Autodesk Inventor part; units mm, degrees
(part 2 of 2)
  spline S27 degree 3 poles (-6.8794, 42.2876) (-6.8611, 42.277) (-6.8428, 42.2665) (-6.8244, 42.2562) (-6.7977, 42.2413) (-6.7709, 42.2265) (-6.744, 42.2121) (-6.7179, 42.1982) (-6.6917, 42.1845) (-6.6654, 42.171) (-6.6399, 42.158) (-6.6144, 42.1453) (-6.5887, 42.1329) (-6.5639, 42.1208) (-6.5389, 42.109) (-6.5139, 42.0975) (-6.4898, 42.0864) (-6.4655, 42.0755) (-6.4412, 42.0649) (-6.4178, 42.0547) (-6.3942, 42.0447) (-6.3706, 42.0349) (-6.3479, 42.0255) (-6.3251, 42.0164) (-6.3022, 42.0075) (-6.2803, 41.9989) (-6.2583, 41.9906) (-6.2362, 41.9825) (-6.215, 41.9747) (-6.1937, 41.9671) (-6.1724, 41.9598) (-6.152, 41.9528) (-6.1316, 41.946) (-6.1111, 41.9394) (-6.0915, 41.9331) (-6.0719, 41.9269) (-6.0522, 41.921) (-6.0335, 41.9154) (-6.0147, 41.91) (-5.9959, 41.9047) (-5.978, 41.8998) (-5.9601, 41.895) (-5.9422, 41.8904) (-5.9252, 41.886) (-5.9081, 41.8818) (-5.8911, 41.8778) (-5.875, 41.874) (-5.8588, 41.8703) (-5.8427, 41.8668) (-5.8275, 41.8636) (-5.8123, 41.8605) (-5.797, 41.8575) (-5.7827, 41.8547) (-5.7684, 41.8521) (-5.7541, 41.8496) (-5.7408, 41.8473) (-5.7274, 41.8451) (-5.7141, 41.8431) (-5.7017, 41.8412) (-5.6893, 41.8394) (-5.6768, 41.8378) (-5.6654, 41.8363) (-5.654, 41.8349) (-5.6425, 41.8336) (-5.6321, 41.8324) (-5.6216, 41.8313) (-5.6111, 41.8304) (-5.6016, 41.8295) (-5.5921, 41.8287) (-5.5826, 41.828) (-5.5741, 41.8274) (-5.5656, 41.8269) (-5.5571, 41.8265) (-5.5496, 41.8261) (-5.5421, 41.8258) (-5.5346, 41.8255) (-5.5231, 41.8252) (-5.5115, 41.825) (-5.5, 41.825) knots 0 0 0 0 0.043076 0.043076 0.043076 0.105506 0.105506 0.105506 0.165888 0.165888 0.165888 0.224224 0.224224 0.224224 0.280513 0.280513 0.280513 0.334755 0.334755 0.334755 0.38695 0.38695 0.38695 0.437099 0.437099 0.437099 0.4852 0.4852 0.4852 0.531254 0.531254 0.531254 0.575262 0.575262 0.575262 0.617223 0.617223 0.617223 0.657137 0.657137 0.657137 0.695004 0.695004 0.695004 0.730824 0.730824 0.730824 0.764598 0.764598 0.764598 0.796324 0.796324 0.796324 0.826004 0.826004 0.826004 0.853636 0.853636 0.853636 0.879222 0.879222 0.879222 0.902761 0.902761 0.902761 0.924253 0.924253 0.924253 0.943699 0.943699 0.943699 0.961097 0.961097 0.961097 0.976448 0.976448 0.976448 1 1 1 1
  line L41 (-5.5, 41.825) -> (-4.55, 41.825)
  line L42 (-4.55, 44.961) -> (-4.55, 46.5908)
  line L43 (-4.55, 46.5908) -> (-5.5, 46.5908)
  spline S28 degree 3 poles (-5.5, 46.5908) (-5.5115, 46.5908) (-5.5306, 46.5905) (-5.5581, 46.5893) (-5.5836, 46.5877) (-5.6121, 46.5854) (-5.6435, 46.5822) (-5.6779, 46.578) (-5.7151, 46.5726) (-5.7551, 46.5661) (-5.798, 46.5582) (-5.8437, 46.5489) (-5.8921, 46.5379) (-5.9432, 46.5253) (-5.9969, 46.5109) (-6.0532, 46.4946) (-6.1121, 46.4763) (-6.1734, 46.4558) (-6.2372, 46.4332) (-6.3033, 46.4081) (-6.3716, 46.3807) (-6.4422, 46.3507) (-6.5149, 46.3181) (-6.5897, 46.2827) (-6.6664, 46.2445) (-6.745, 46.2034) (-6.8162, 46.1644) (-6.8611, 46.1388) (-6.8794, 46.1282) knots 0 0 0 0 0.023552 0.038904 0.056302 0.075747 0.097239 0.120778 0.146364 0.173997 0.203676 0.235403 0.269176 0.304996 0.342863 0.382777 0.424738 0.468746 0.5148 0.562902 0.61305 0.665245 0.719487 0.775776 0.834112 0.894494 0.956924 1 1 1 1
  arc A14 (-6.8794, 46.1282) -> (-6.8794, 45.4236) centre (2.0124, 45.7759) ccw
  spline S29 degree 3 poles (-6.8794, 45.4236) (-6.8611, 45.413) (-6.8428, 45.4025) (-6.8244, 45.3922) (-6.7977, 45.3773) (-6.7709, 45.3625) (-6.744, 45.3481) (-6.7179, 45.3342) (-6.6917, 45.3205) (-6.6654, 45.307) (-6.6399, 45.294) (-6.6144, 45.2813) (-6.5887, 45.2689) (-6.5639, 45.2568) (-6.5389, 45.245) (-6.5139, 45.2335) (-6.4898, 45.2224) (-6.4655, 45.2115) (-6.4412, 45.2009) (-6.4178, 45.1907) (-6.3942, 45.1807) (-6.3706, 45.1709) (-6.3479, 45.1615) (-6.3251, 45.1524) (-6.3022, 45.1435) (-6.2803, 45.1349) (-6.2583, 45.1266) (-6.2362, 45.1185) (-6.215, 45.1107) (-6.1937, 45.1031) (-6.1724, 45.0958) (-6.152, 45.0888) (-6.1316, 45.082) (-6.1111, 45.0754) (-6.0915, 45.0691) (-6.0719, 45.0629) (-6.0522, 45.057) (-6.0335, 45.0514) (-6.0147, 45.046) (-5.9959, 45.0407) (-5.978, 45.0358) (-5.9601, 45.031) (-5.9422, 45.0264) (-5.9252, 45.022) (-5.9081, 45.0178) (-5.8911, 45.0138) (-5.875, 45.01) (-5.8588, 45.0063) (-5.8427, 45.0028) (-5.8275, 44.9996) (-5.8123, 44.9965) (-5.797, 44.9935) (-5.7827, 44.9907) (-5.7684, 44.9881) (-5.7541, 44.9856) (-5.7408, 44.9833) (-5.7274, 44.9811) (-5.7141, 44.9791) (-5.7017, 44.9772) (-5.6893, 44.9754) (-5.6768, 44.9738) (-5.6654, 44.9723) (-5.654, 44.9709) (-5.6425, 44.9696) (-5.6321, 44.9684) (-5.6216, 44.9673) (-5.6111, 44.9664) (-5.6016, 44.9655) (-5.5921, 44.9647) (-5.5826, 44.964) (-5.5741, 44.9634) (-5.5656, 44.9629) (-5.5571, 44.9625) (-5.5496, 44.9621) (-5.5421, 44.9618) (-5.5346, 44.9615) (-5.5231, 44.9612) (-5.5115, 44.961) (-5.5, 44.961) knots 0 0 0 0 0.043076 0.043076 0.043076 0.105506 0.105506 0.105506 0.165888 0.165888 0.165888 0.224224 0.224224 0.224224 0.280513 0.280513 0.280513 0.334755 0.334755 0.334755 0.38695 0.38695 0.38695 0.437099 0.437099 0.437099 0.4852 0.4852 0.4852 0.531254 0.531254 0.531254 0.575262 0.575262 0.575262 0.617223 0.617223 0.617223 0.657137 0.657137 0.657137 0.695004 0.695004 0.695004 0.730824 0.730824 0.730824 0.764598 0.764598 0.764598 0.796324 0.796324 0.796324 0.826004 0.826004 0.826004 0.853636 0.853636 0.853636 0.879222 0.879222 0.879222 0.902761 0.902761 0.902761 0.924253 0.924253 0.924253 0.943699 0.943699 0.943699 0.961097 0.961097 0.961097 0.976448 0.976448 0.976448 1 1 1 1
  line L44 (-5.5, 44.961) -> (-4.55, 44.961)
  line L45 (-4.55, 48.097) -> (-4.55, 49.7268)
  line L46 (-4.55, 49.7268) -> (-5.5, 49.7268)
  spline S30 degree 3 poles (-5.5, 49.7268) (-5.5115, 49.7268) (-5.5306, 49.7265) (-5.5581, 49.7253) (-5.5836, 49.7237) (-5.6121, 49.7214) (-5.6435, 49.7182) (-5.6779, 49.714) (-5.7151, 49.7086) (-5.7551, 49.7021) (-5.798, 49.6942) (-5.8437, 49.6849) (-5.8921, 49.6739) (-5.9432, 49.6613) (-5.9969, 49.6469) (-6.0532, 49.6306) (-6.1121, 49.6123) (-6.1734, 49.5918) (-6.2372, 49.5692) (-6.3033, 49.5441) (-6.3716, 49.5167) (-6.4422, 49.4867) (-6.5149, 49.4541) (-6.5897, 49.4187) (-6.6664, 49.3805) (-6.745, 49.3394) (-6.8162, 49.3004) (-6.8611, 49.2748) (-6.8794, 49.2642) knots 0 0 0 0 0.023552 0.038904 0.056302 0.075747 0.097239 0.120778 0.146364 0.173997 0.203676 0.235403 0.269176 0.304996 0.342863 0.382777 0.424738 0.468746 0.5148 0.562902 0.61305 0.665245 0.719487 0.775776 0.834112 0.894494 0.956924 1 1 1 1
  arc A15 (-6.8794, 49.2642) -> (-6.8794, 48.5596) centre (2.0124, 48.9119) ccw
  spline S31 degree 3 poles (-6.8794, 48.5596) (-6.8611, 48.549) (-6.8428, 48.5385) (-6.8244, 48.5282) (-6.7977, 48.5133) (-6.7709, 48.4985) (-6.744, 48.4841) (-6.7179, 48.4702) (-6.6917, 48.4565) (-6.6654, 48.443) (-6.6399, 48.43) (-6.6144, 48.4173) (-6.5887, 48.4049) (-6.5639, 48.3928) (-6.5389, 48.381) (-6.5139, 48.3695) (-6.4898, 48.3584) (-6.4655, 48.3475) (-6.4412, 48.3369) (-6.4178, 48.3267) (-6.3942, 48.3167) (-6.3706, 48.3069) (-6.3479, 48.2975) (-6.3251, 48.2884) (-6.3022, 48.2795) (-6.2803, 48.2709) (-6.2583, 48.2626) (-6.2362, 48.2545) (-6.215, 48.2467) (-6.1937, 48.2391) (-6.1724, 48.2318) (-6.152, 48.2248) (-6.1316, 48.218) (-6.1111, 48.2114) (-6.0915, 48.2051) (-6.0719, 48.1989) (-6.0522, 48.193) (-6.0335, 48.1874) (-6.0147, 48.182) (-5.9959, 48.1767) (-5.978, 48.1718) (-5.9601, 48.167) (-5.9422, 48.1624) (-5.9252, 48.158) (-5.9081, 48.1538) (-5.8911, 48.1498) (-5.875, 48.146) (-5.8588, 48.1423) (-5.8427, 48.1388) (-5.8275, 48.1356) (-5.8123, 48.1325) (-5.797, 48.1295) (-5.7827, 48.1267) (-5.7684, 48.1241) (-5.7541, 48.1216) (-5.7408, 48.1193) (-5.7274, 48.1171) (-5.7141, 48.1151) (-5.7017, 48.1132) (-5.6893, 48.1114) (-5.6768, 48.1098) (-5.6654, 48.1083) (-5.654, 48.1069) (-5.6425, 48.1056) (-5.6321, 48.1044) (-5.6216, 48.1033) (-5.6111, 48.1024) (-5.6016, 48.1015) (-5.5921, 48.1007) (-5.5826, 48.1) (-5.5741, 48.0994) (-5.5656, 48.0989) (-5.5571, 48.0985) (-5.5496, 48.0981) (-5.5421, 48.0978) (-5.5346, 48.0975) (-5.5231, 48.0972) (-5.5115, 48.097) (-5.5, 48.097) knots 0 0 0 0 0.043076 0.043076 0.043076 0.105506 0.105506 0.105506 0.165888 0.165888 0.165888 0.224224 0.224224 0.224224 0.280513 0.280513 0.280513 0.334755 0.334755 0.334755 0.38695 0.38695 0.38695 0.437099 0.437099 0.437099 0.4852 0.4852 0.4852 0.531254 0.531254 0.531254 0.575262 0.575262 0.575262 0.617223 0.617223 0.617223 0.657137 0.657137 0.657137 0.695004 0.695004 0.695004 0.730824 0.730824 0.730824 0.764598 0.764598 0.764598 0.796324 0.796324 0.796324 0.826004 0.826004 0.826004 0.853636 0.853636 0.853636 0.879222 0.879222 0.879222 0.902761 0.902761 0.902761 0.924253 0.924253 0.924253 0.943699 0.943699 0.943699 0.961097 0.961097 0.961097 0.976448 0.976448 0.976448 1 1 1 1
  line L47 (-5.5, 48.097) -> (-4.55, 48.097)
  line L48 (-4.55, 51.233) -> (-4.55, 52.8628)
  line L49 (-4.55, 52.8628) -> (-5.5, 52.8628)
  spline S32 degree 3 poles (-5.5, 52.8628) (-5.5115, 52.8628) (-5.5306, 52.8625) (-5.5581, 52.8613) (-5.5836, 52.8597) (-5.6121, 52.8574) (-5.6435, 52.8542) (-5.6779, 52.85) (-5.7151, 52.8446) (-5.7551, 52.8381) (-5.798, 52.8302) (-5.8437, 52.8209) (-5.8921, 52.8099) (-5.9432, 52.7973) (-5.9969, 52.7829) (-6.0532, 52.7666) (-6.1121, 52.7483) (-6.1734, 52.7278) (-6.2372, 52.7052) (-6.3033, 52.6801) (-6.3716, 52.6527) (-6.4422, 52.6227) (-6.5149, 52.5901) (-6.5897, 52.5547) (-6.6664, 52.5165) (-6.745, 52.4754) (-6.8162, 52.4364) (-6.8611, 52.4108) (-6.8794, 52.4002) knots 0 0 0 0 0.023552 0.038904 0.056302 0.075747 0.097239 0.120778 0.146364 0.173997 0.203676 0.235403 0.269176 0.304996 0.342863 0.382777 0.424738 0.468746 0.5148 0.562902 0.61305 0.665245 0.719487 0.775776 0.834112 0.894494 0.956924 1 1 1 1
  arc A16 (-6.8794, 52.4002) -> (-6.8794, 51.6956) centre (2.0124, 52.0479) ccw
  spline S33 degree 3 poles (-6.8794, 51.6956) (-6.8611, 51.685) (-6.8428, 51.6745) (-6.8244, 51.6642) (-6.7977, 51.6493) (-6.7709, 51.6345) (-6.744, 51.6201) (-6.7179, 51.6062) (-6.6917, 51.5925) (-6.6654, 51.579) (-6.6399, 51.566) (-6.6144, 51.5533) (-6.5887, 51.5409) (-6.5639, 51.5288) (-6.5389, 51.517) (-6.5139, 51.5055) (-6.4898, 51.4944) (-6.4655, 51.4835) (-6.4412, 51.4729) (-6.4178, 51.4627) (-6.3942, 51.4527) (-6.3706, 51.4429) (-6.3479, 51.4335) (-6.3251, 51.4244) (-6.3022, 51.4155) (-6.2803, 51.4069) (-6.2583, 51.3986) (-6.2362, 51.3905) (-6.215, 51.3827) (-6.1937, 51.3751) (-6.1724, 51.3678) (-6.152, 51.3608) (-6.1316, 51.354) (-6.1111, 51.3474) (-6.0915, 51.3411) (-6.0719, 51.3349) (-6.0522, 51.329) (-6.0335, 51.3234) (-6.0147, 51.318) (-5.9959, 51.3127) (-5.978, 51.3078) (-5.9601, 51.303) (-5.9422, 51.2984) (-5.9252, 51.294) (-5.9081, 51.2898) (-5.8911, 51.2858) (-5.875, 51.282) (-5.8588, 51.2783) (-5.8427, 51.2748) (-5.8275, 51.2716) (-5.8123, 51.2685) (-5.797, 51.2655) (-5.7827, 51.2627) (-5.7684, 51.2601) (-5.7541, 51.2576) (-5.7408, 51.2553) (-5.7274, 51.2531) (-5.7141, 51.2511) (-5.7017, 51.2492) (-5.6893, 51.2474) (-5.6768, 51.2458) (-5.6654, 51.2443) (-5.654, 51.2429) (-5.6425, 51.2416) (-5.6321, 51.2404) (-5.6216, 51.2393) (-5.6111, 51.2384) (-5.6016, 51.2375) (-5.5921, 51.2367) (-5.5826, 51.236) (-5.5741, 51.2354) (-5.5656, 51.2349) (-5.5571, 51.2345) (-5.5496, 51.2341) (-5.5421, 51.2338) (-5.5346, 51.2335) (-5.5231, 51.2332) (-5.5115, 51.233) (-5.5, 51.233) knots 0 0 0 0 0.043076 0.043076 0.043076 0.105506 0.105506 0.105506 0.165888 0.165888 0.165888 0.224224 0.224224 0.224224 0.280513 0.280513 0.280513 0.334755 0.334755 0.334755 0.38695 0.38695 0.38695 0.437099 0.437099 0.437099 0.4852 0.4852 0.4852 0.531254 0.531254 0.531254 0.575262 0.575262 0.575262 0.617223 0.617223 0.617223 0.657137 0.657137 0.657137 0.695004 0.695004 0.695004 0.730824 0.730824 0.730824 0.764598 0.764598 0.764598 0.796324 0.796324 0.796324 0.826004 0.826004 0.826004 0.853636 0.853636 0.853636 0.879222 0.879222 0.879222 0.902761 0.902761 0.902761 0.924253 0.924253 0.924253 0.943699 0.943699 0.943699 0.961097 0.961097 0.961097 0.976448 0.976448 0.976448 1 1 1 1
  line L50 (-5.5, 51.233) -> (-4.55, 51.233)
  line L51 (-4.55, 54.369) -> (-4.55, 55.9988)
  line L52 (-4.55, 55.9988) -> (-5.5, 55.9988)
  spline S34 degree 3 poles (-5.5, 55.9988) (-5.5115, 55.9988) (-5.5306, 55.9985) (-5.5581, 55.9973) (-5.5836, 55.9957) (-5.6121, 55.9934) (-5.6435, 55.9902) (-5.6779, 55.986) (-5.7151, 55.9806) (-5.7551, 55.9741) (-5.798, 55.9662) (-5.8437, 55.9569) (-5.8921, 55.9459) (-5.9432, 55.9333) (-5.9969, 55.9189) (-6.0532, 55.9026) (-6.1121, 55.8843) (-6.1734, 55.8638) (-6.2372, 55.8412) (-6.3033, 55.8161) (-6.3716, 55.7887) (-6.4422, 55.7587) (-6.5149, 55.7261) (-6.5897, 55.6907) (-6.6664, 55.6525) (-6.745, 55.6114) (-6.8162, 55.5724) (-6.8611, 55.5468) (-6.8794, 55.5362) knots 0 0 0 0 0.023552 0.038904 0.056302 0.075747 0.097239 0.120778 0.146364 0.173997 0.203676 0.235403 0.269176 0.304996 0.342863 0.382777 0.424738 0.468746 0.5148 0.562902 0.61305 0.665245 0.719487 0.775776 0.834112 0.894494 0.956924 1 1 1 1
  arc A17 (-6.8794, 55.5362) -> (-6.8794, 54.8316) centre (2.0124, 55.1839) ccw
  spline S35 degree 3 poles (-6.8794, 54.8316) (-6.8611, 54.821) (-6.8428, 54.8105) (-6.8244, 54.8002) (-6.7977, 54.7853) (-6.7709, 54.7705) (-6.744, 54.7561) (-6.7179, 54.7422) (-6.6917, 54.7285) (-6.6654, 54.715) (-6.6399, 54.702) (-6.6144, 54.6893) (-6.5887, 54.6769) (-6.5639, 54.6648) (-6.5389, 54.653) (-6.5139, 54.6415) (-6.4898, 54.6304) (-6.4655, 54.6195) (-6.4412, 54.6089) (-6.4178, 54.5987) (-6.3942, 54.5887) (-6.3706, 54.5789) (-6.3479, 54.5695) (-6.3251, 54.5604) (-6.3022, 54.5515) (-6.2803, 54.5429) (-6.2583, 54.5346) (-6.2362, 54.5265) (-6.215, 54.5187) (-6.1937, 54.5111) (-6.1724, 54.5038) (-6.152, 54.4968) (-6.1316, 54.49) (-6.1111, 54.4834) (-6.0915, 54.4771) (-6.0719, 54.4709) (-6.0522, 54.465) (-6.0335, 54.4594) (-6.0147, 54.454) (-5.9959, 54.4487) (-5.978, 54.4438) (-5.9601, 54.439) (-5.9422, 54.4344) (-5.9252, 54.43) (-5.9081, 54.4258) (-5.8911, 54.4218) (-5.875, 54.418) (-5.8588, 54.4143) (-5.8427, 54.4108) (-5.8275, 54.4076) (-5.8123, 54.4045) (-5.797, 54.4015) (-5.7827, 54.3987) (-5.7684, 54.3961) (-5.7541, 54.3936) (-5.7408, 54.3913) (-5.7274, 54.3891) (-5.7141, 54.3871) (-5.7017, 54.3852) (-5.6893, 54.3834) (-5.6768, 54.3818) (-5.6654, 54.3803) (-5.654, 54.3789) (-5.6425, 54.3776) (-5.6321, 54.3764) (-5.6216, 54.3753) (-5.6111, 54.3744) (-5.6016, 54.3735) (-5.5921, 54.3727) (-5.5826, 54.372) (-5.5741, 54.3714) (-5.5656, 54.3709) (-5.5571, 54.3705) (-5.5496, 54.3701) (-5.5421, 54.3698) (-5.5346, 54.3695) (-5.5231, 54.3692) (-5.5115, 54.369) (-5.5, 54.369) knots 0 0 0 0 0.043076 0.043076 0.043076 0.105506 0.105506 0.105506 0.165888 0.165888 0.165888 0.224224 0.224224 0.224224 0.280513 0.280513 0.280513 0.334755 0.334755 0.334755 0.38695 0.38695 0.38695 0.437099 0.437099 0.437099 0.4852 0.4852 0.4852 0.531254 0.531254 0.531254 0.575262 0.575262 0.575262 0.617223 0.617223 0.617223 0.657137 0.657137 0.657137 0.695004 0.695004 0.695004 0.730824 0.730824 0.730824 0.764598 0.764598 0.764598 0.796324 0.796324 0.796324 0.826004 0.826004 0.826004 0.853636 0.853636 0.853636 0.879222 0.879222 0.879222 0.902761 0.902761 0.902761 0.924253 0.924253 0.924253 0.943699 0.943699 0.943699 0.961097 0.961097 0.961097 0.976448 0.976448 0.976448 1 1 1 1
  line L53 (-5.5, 54.369) -> (-4.55, 54.369)
  line L54 (-4.55, 57.505) -> (-4.55, 59.1348)
  line L55 (-4.55, 59.1348) -> (-5.5, 59.1348)
  spline S36 degree 3 poles (-5.5, 59.1348) (-5.5115, 59.1348) (-5.5306, 59.1345) (-5.5581, 59.1333) (-5.5836, 59.1317) (-5.6121, 59.1294) (-5.6435, 59.1262) (-5.6779, 59.122) (-5.7151, 59.1166) (-5.7551, 59.1101) (-5.798, 59.1022) (-5.8437, 59.0929) (-5.8921, 59.0819) (-5.9432, 59.0693) (-5.9969, 59.0549) (-6.0532, 59.0386) (-6.1121, 59.0203) (-6.1734, 58.9998) (-6.2372, 58.9772) (-6.3033, 58.9521) (-6.3716, 58.9247) (-6.4422, 58.8947) (-6.5149, 58.8621) (-6.5897, 58.8267) (-6.6664, 58.7885) (-6.745, 58.7474) (-6.8162, 58.7084) (-6.8611, 58.6828) (-6.8794, 58.6722) knots 0 0 0 0 0.023552 0.038904 0.056302 0.075747 0.097239 0.120778 0.146364 0.173997 0.203676 0.235403 0.269176 0.304996 0.342863 0.382777 0.424738 0.468746 0.5148 0.562902 0.61305 0.665245 0.719487 0.775776 0.834112 0.894494 0.956924 1 1 1 1
  arc A18 (-6.8794, 58.6722) -> (-6.8794, 57.9676) centre (2.0124, 58.3199) ccw
  spline S37 degree 3 poles (-6.8794, 57.9676) (-6.8611, 57.957) (-6.8428, 57.9465) (-6.8244, 57.9362) (-6.7977, 57.9213) (-6.7709, 57.9065) (-6.744, 57.8921) (-6.7179, 57.8782) (-6.6917, 57.8645) (-6.6654, 57.851) (-6.6399, 57.838) (-6.6144, 57.8253) (-6.5887, 57.8129) (-6.5639, 57.8008) (-6.5389, 57.789) (-6.5139, 57.7775) (-6.4898, 57.7664) (-6.4655, 57.7555) (-6.4412, 57.7449) (-6.4178, 57.7347) (-6.3942, 57.7247) (-6.3706, 57.7149) (-6.3479, 57.7055) (-6.3251, 57.6964) (-6.3022, 57.6875) (-6.2803, 57.6789) (-6.2583, 57.6706) (-6.2362, 57.6625) (-6.215, 57.6547) (-6.1937, 57.6471) (-6.1724, 57.6398) (-6.152, 57.6328) (-6.1316, 57.626) (-6.1111, 57.6194) (-6.0915, 57.6131) (-6.0719, 57.6069) (-6.0522, 57.601) (-6.0335, 57.5954) (-6.0147, 57.59) (-5.9959, 57.5847) (-5.978, 57.5798) (-5.9601, 57.575) (-5.9422, 57.5704) (-5.9252, 57.566) (-5.9081, 57.5618) (-5.8911, 57.5578) (-5.875, 57.554) (-5.8588, 57.5503) (-5.8427, 57.5468) (-5.8275, 57.5436) (-5.8123, 57.5405) (-5.797, 57.5375) (-5.7827, 57.5347) (-5.7684, 57.5321) (-5.7541, 57.5296) (-5.7408, 57.5273) (-5.7274, 57.5251) (-5.7141, 57.5231) (-5.7017, 57.5212) (-5.6893, 57.5194) (-5.6768, 57.5178) (-5.6654, 57.5163) (-5.654, 57.5149) (-5.6425, 57.5136) (-5.6321, 57.5124) (-5.6216, 57.5113) (-5.6111, 57.5104) (-5.6016, 57.5095) (-5.5921, 57.5087) (-5.5826, 57.508) (-5.5741, 57.5074) (-5.5656, 57.5069) (-5.5571, 57.5065) (-5.5496, 57.5061) (-5.5421, 57.5058) (-5.5346, 57.5055) (-5.5231, 57.5052) (-5.5115, 57.505) (-5.5, 57.505) knots 0 0 0 0 0.043076 0.043076 0.043076 0.105506 0.105506 0.105506 0.165888 0.165888 0.165888 0.224224 0.224224 0.224224 0.280513 0.280513 0.280513 0.334755 0.334755 0.334755 0.38695 0.38695 0.38695 0.437099 0.437099 0.437099 0.4852 0.4852 0.4852 0.531254 0.531254 0.531254 0.575262 0.575262 0.575262 0.617223 0.617223 0.617223 0.657137 0.657137 0.657137 0.695004 0.695004 0.695004 0.730824 0.730824 0.730824 0.764598 0.764598 0.764598 0.796324 0.796324 0.796324 0.826004 0.826004 0.826004 0.853636 0.853636 0.853636 0.879222 0.879222 0.879222 0.902761 0.902761 0.902761 0.924253 0.924253 0.924253 0.943699 0.943699 0.943699 0.961097 0.961097 0.961097 0.976448 0.976448 0.976448 1 1 1 1
  line L56 (-5.5, 57.505) -> (-4.55, 57.505)
  line L57 (-4.55, 60.641) -> (-4.55, 62.2708)
  line L58 (-4.55, 62.2708) -> (-5.5, 62.2708)
  spline S38 degree 3 poles (-5.5, 62.2708) (-5.5115, 62.2708) (-5.5306, 62.2705) (-5.5581, 62.2693) (-5.5836, 62.2677) (-5.6121, 62.2654) (-5.6435, 62.2622) (-5.6779, 62.258) (-5.7151, 62.2526) (-5.7551, 62.2461) (-5.798, 62.2382) (-5.8437, 62.2289) (-5.8921, 62.2179) (-5.9432, 62.2053) (-5.9969, 62.1909) (-6.0532, 62.1746) (-6.1121, 62.1563) (-6.1734, 62.1358) (-6.2372, 62.1132) (-6.3033, 62.0881) (-6.3716, 62.0607) (-6.4422, 62.0307) (-6.5149, 61.9981) (-6.5897, 61.9627) (-6.6664, 61.9245) (-6.745, 61.8834) (-6.8162, 61.8444) (-6.8611, 61.8188) (-6.8794, 61.8082) knots 0 0 0 0 0.023552 0.038904 0.056302 0.075747 0.097239 0.120778 0.146364 0.173997 0.203676 0.235403 0.269176 0.304996 0.342863 0.382777 0.424738 0.468746 0.5148 0.562902 0.61305 0.665245 0.719487 0.775776 0.834112 0.894494 0.956924 1 1 1 1
  arc A19 (-6.8794, 61.8082) -> (-6.8794, 61.1036) centre (2.0124, 61.4559) ccw
  spline S39 degree 3 poles (-6.8794, 61.1036) (-6.8611, 61.093) (-6.8428, 61.0825) (-6.8244, 61.0722) (-6.7977, 61.0573) (-6.7709, 61.0425) (-6.744, 61.0281) (-6.7179, 61.0142) (-6.6917, 61.0005) (-6.6654, 60.987) (-6.6399, 60.974) (-6.6144, 60.9613) (-6.5887, 60.9489) (-6.5639, 60.9368) (-6.5389, 60.925) (-6.5139, 60.9135) (-6.4898, 60.9024) (-6.4655, 60.8915) (-6.4412, 60.8809) (-6.4178, 60.8707) (-6.3942, 60.8607) (-6.3706, 60.8509) (-6.3479, 60.8415) (-6.3251, 60.8324) (-6.3022, 60.8235) (-6.2803, 60.8149) (-6.2583, 60.8066) (-6.2362, 60.7985) (-6.215, 60.7907) (-6.1937, 60.7831) (-6.1724, 60.7758) (-6.152, 60.7688) (-6.1316, 60.762) (-6.1111, 60.7554) (-6.0915, 60.7491) (-6.0719, 60.7429) (-6.0522, 60.737) (-6.0335, 60.7314) (-6.0147, 60.726) (-5.9959, 60.7207) (-5.978, 60.7158) (-5.9601, 60.711) (-5.9422, 60.7064) (-5.9252, 60.702) (-5.9081, 60.6978) (-5.8911, 60.6938) (-5.875, 60.69) (-5.8588, 60.6863) (-5.8427, 60.6828) (-5.8275, 60.6796) (-5.8123, 60.6765) (-5.797, 60.6735) (-5.7827, 60.6707) (-5.7684, 60.6681) (-5.7541, 60.6656) (-5.7408, 60.6633) (-5.7274, 60.6611) (-5.7141, 60.6591) (-5.7017, 60.6572) (-5.6893, 60.6554) (-5.6768, 60.6538) (-5.6654, 60.6523) (-5.654, 60.6509) (-5.6425, 60.6496) (-5.6321, 60.6484) (-5.6216, 60.6473) (-5.6111, 60.6464) (-5.6016, 60.6455) (-5.5921, 60.6447) (-5.5826, 60.644) (-5.5741, 60.6434) (-5.5656, 60.6429) (-5.5571, 60.6425) (-5.5496, 60.6421) (-5.5421, 60.6418) (-5.5346, 60.6415) (-5.5231, 60.6412) (-5.5115, 60.641) (-5.5, 60.641) knots 0 0 0 0 0.043076 0.043076 0.043076 0.105506 0.105506 0.105506 0.165888 0.165888 0.165888 0.224224 0.224224 0.224224 0.280513 0.280513 0.280513 0.334755 0.334755 0.334755 0.38695 0.38695 0.38695 0.437099 0.437099 0.437099 0.4852 0.4852 0.4852 0.531254 0.531254 0.531254 0.575262 0.575262 0.575262 0.617223 0.617223 0.617223 0.657137 0.657137 0.657137 0.695004 0.695004 0.695004 0.730824 0.730824 0.730824 0.764598 0.764598 0.764598 0.796324 0.796324 0.796324 0.826004 0.826004 0.826004 0.853636 0.853636 0.853636 0.879222 0.879222 0.879222 0.902761 0.902761 0.902761 0.924253 0.924253 0.924253 0.943699 0.943699 0.943699 0.961097 0.961097 0.961097 0.976448 0.976448 0.976448 1 1 1 1
  line L59 (-5.5, 60.641) -> (-4.55, 60.641)
  line L60 (-4.55, 63.777) -> (-4.55, 65.4068)
  line L61 (-4.55, 65.4068) -> (-5.5, 65.4068)
  spline S40 degree 3 poles (-5.5, 65.4068) (-5.5115, 65.4068) (-5.5306, 65.4065) (-5.5581, 65.4053) (-5.5836, 65.4037) (-5.6121, 65.4014) (-5.6435, 65.3982) (-5.6779, 65.394) (-5.7151, 65.3886) (-5.7551, 65.3821) (-5.798, 65.3742) (-5.8437, 65.3649) (-5.8921, 65.3539) (-5.9432, 65.3413) (-5.9969, 65.3269) (-6.0532, 65.3106) (-6.1121, 65.2923) (-6.1734, 65.2718) (-6.2372, 65.2492) (-6.3033, 65.2241) (-6.3716, 65.1967) (-6.4422, 65.1667) (-6.5149, 65.1341) (-6.5897, 65.0987) (-6.6664, 65.0605) (-6.745, 65.0194) (-6.8162, 64.9804) (-6.8611, 64.9548) (-6.8794, 64.9442) knots 0 0 0 0 0.023552 0.038904 0.056302 0.075747 0.097239 0.120778 0.146364 0.173997 0.203676 0.235403 0.269176 0.304996 0.342863 0.382777 0.424738 0.468746 0.5148 0.562902 0.61305 0.665245 0.719487 0.775776 0.834112 0.894494 0.956924 1 1 1 1
  arc A20 (-6.8794, 64.9442) -> (-6.8794, 64.2396) centre (2.0124, 64.5919) ccw
  spline S41 degree 3 poles (-6.8794, 64.2396) (-6.8611, 64.229) (-6.8428, 64.2185) (-6.8244, 64.2082) (-6.7977, 64.1933) (-6.7709, 64.1785) (-6.744, 64.1641) (-6.7179, 64.1502) (-6.6917, 64.1365) (-6.6654, 64.123) (-6.6399, 64.11) (-6.6144, 64.0973) (-6.5887, 64.0849) (-6.5639, 64.0728) (-6.5389, 64.061) (-6.5139, 64.0495) (-6.4898, 64.0384) (-6.4655, 64.0275) (-6.4412, 64.0169) (-6.4178, 64.0067) (-6.3942, 63.9967) (-6.3706, 63.9869) (-6.3479, 63.9775) (-6.3251, 63.9684) (-6.3022, 63.9595) (-6.2803, 63.9509) (-6.2583, 63.9426) (-6.2362, 63.9345) (-6.215, 63.9267) (-6.1937, 63.9191) (-6.1724, 63.9118) (-6.152, 63.9048) (-6.1316, 63.898) (-6.1111, 63.8914) (-6.0915, 63.8851) (-6.0719, 63.8789) (-6.0522, 63.873) (-6.0335, 63.8674) (-6.0147, 63.862) (-5.9959, 63.8567) (-5.978, 63.8518) (-5.9601, 63.847) (-5.9422, 63.8424) (-5.9252, 63.838) (-5.9081, 63.8338) (-5.8911, 63.8298) (-5.875, 63.826) (-5.8588, 63.8223) (-5.8427, 63.8188) (-5.8275, 63.8156) (-5.8123, 63.8125) (-5.797, 63.8095) (-5.7827, 63.8067) (-5.7684, 63.8041) (-5.7541, 63.8016) (-5.7408, 63.7993) (-5.7274, 63.7971) (-5.7141, 63.7951) (-5.7017, 63.7932) (-5.6893, 63.7914) (-5.6768, 63.7898) (-5.6654, 63.7883) (-5.654, 63.7869) (-5.6425, 63.7856) (-5.6321, 63.7844) (-5.6216, 63.7833) (-5.6111, 63.7824) (-5.6016, 63.7815) (-5.5921, 63.7807) (-5.5826, 63.78) (-5.5741, 63.7794) (-5.5656, 63.7789) (-5.5571, 63.7785) (-5.5496, 63.7781) (-5.5421, 63.7778) (-5.5346, 63.7775) (-5.5231, 63.7772) (-5.5115, 63.777) (-5.5, 63.777) knots 0 0 0 0 0.043076 0.043076 0.043076 0.105506 0.105506 0.105506 0.165888 0.165888 0.165888 0.224224 0.224224 0.224224 0.280513 0.280513 0.280513 0.334755 0.334755 0.334755 0.38695 0.38695 0.38695 0.437099 0.437099 0.437099 0.4852 0.4852 0.4852 0.531254 0.531254 0.531254 0.575262 0.575262 0.575262 0.617223 0.617223 0.617223 0.657137 0.657137 0.657137 0.695004 0.695004 0.695004 0.730824 0.730824 0.730824 0.764598 0.764598 0.764598 0.796324 0.796324 0.796324 0.826004 0.826004 0.826004 0.853636 0.853636 0.853636 0.879222 0.879222 0.879222 0.902761 0.902761 0.902761 0.924253 0.924253 0.924253 0.943699 0.943699 0.943699 0.961097 0.961097 0.961097 0.976448 0.976448 0.976448 1 1 1 1
  line L62 (-5.5, 63.777) -> (-4.55, 63.777)
  line L63 (-4.55, 66.913) -> (-4.55, 68.5428)
  line L64 (-4.55, 68.5428) -> (-5.5, 68.5428)
  spline S42 degree 3 poles (-5.5, 68.5428) (-5.5115, 68.5428) (-5.5306, 68.5425) (-5.5581, 68.5413) (-5.5836, 68.5397) (-5.6121, 68.5374) (-5.6435, 68.5342) (-5.6779, 68.53) (-5.7151, 68.5246) (-5.7551, 68.5181) (-5.798, 68.5102) (-5.8437, 68.5009) (-5.8921, 68.4899) (-5.9432, 68.4773) (-5.9969, 68.4629) (-6.0532, 68.4466) (-6.1121, 68.4283) (-6.1734, 68.4078) (-6.2372, 68.3852) (-6.3033, 68.3601) (-6.3716, 68.3327) (-6.4422, 68.3027) (-6.5149, 68.2701) (-6.5897, 68.2347) (-6.6664, 68.1965) (-6.745, 68.1554) (-6.8162, 68.1164) (-6.8611, 68.0908) (-6.8794, 68.0802) knots 0 0 0 0 0.023552 0.038904 0.056302 0.075747 0.097239 0.120778 0.146364 0.173997 0.203676 0.235403 0.269176 0.304996 0.342863 0.382777 0.424738 0.468746 0.5148 0.562902 0.61305 0.665245 0.719487 0.775776 0.834112 0.894494 0.956924 1 1 1 1
  arc A21 (-6.8794, 68.0802) -> (-6.8794, 67.3756) centre (2.0124, 67.7279) ccw
  spline S43 degree 3 poles (-6.8794, 67.3756) (-6.8611, 67.365) (-6.8428, 67.3545) (-6.8244, 67.3442) (-6.7977, 67.3293) (-6.7709, 67.3145) (-6.744, 67.3001) (-6.7179, 67.2862) (-6.6917, 67.2725) (-6.6654, 67.259) (-6.6399, 67.246) (-6.6144, 67.2333) (-6.5887, 67.2209) (-6.5639, 67.2088) (-6.5389, 67.197) (-6.5139, 67.1855) (-6.4898, 67.1744) (-6.4655, 67.1635) (-6.4412, 67.1529) (-6.4178, 67.1427) (-6.3942, 67.1327) (-6.3706, 67.1229) (-6.3479, 67.1135) (-6.3251, 67.1044) (-6.3022, 67.0955) (-6.2803, 67.0869) (-6.2583, 67.0786) (-6.2362, 67.0705) (-6.215, 67.0627) (-6.1937, 67.0551) (-6.1724, 67.0478) (-6.152, 67.0408) (-6.1316, 67.034) (-6.1111, 67.0274) (-6.0915, 67.0211) (-6.0719, 67.0149) (-6.0522, 67.009) (-6.0335, 67.0034) (-6.0147, 66.998) (-5.9959, 66.9927) (-5.978, 66.9878) (-5.9601, 66.983) (-5.9422, 66.9784) (-5.9252, 66.974) (-5.9081, 66.9698) (-5.8911, 66.9658) (-5.875, 66.962) (-5.8588, 66.9583) (-5.8427, 66.9548) (-5.8275, 66.9516) (-5.8123, 66.9485) (-5.797, 66.9455) (-5.7827, 66.9427) (-5.7684, 66.9401) (-5.7541, 66.9376) (-5.7408, 66.9353) (-5.7274, 66.9331) (-5.7141, 66.9311) (-5.7017, 66.9292) (-5.6893, 66.9274) (-5.6768, 66.9258) (-5.6654, 66.9243) (-5.654, 66.9229) (-5.6425, 66.9216) (-5.6321, 66.9204) (-5.6216, 66.9193) (-5.6111, 66.9184) (-5.6016, 66.9175) (-5.5921, 66.9167) (-5.5826, 66.916) (-5.5741, 66.9154) (-5.5656, 66.9149) (-5.5571, 66.9145) (-5.5496, 66.9141) (-5.5421, 66.9138) (-5.5346, 66.9135) (-5.5231, 66.9132) (-5.5115, 66.913) (-5.5, 66.913) knots 0 0 0 0 0.043076 0.043076 0.043076 0.105506 0.105506 0.105506 0.165888 0.165888 0.165888 0.224224 0.224224 0.224224 0.280513 0.280513 0.280513 0.334755 0.334755 0.334755 0.38695 0.38695 0.38695 0.437099 0.437099 0.437099 0.4852 0.4852 0.4852 0.531254 0.531254 0.531254 0.575262 0.575262 0.575262 0.617223 0.617223 0.617223 0.657137 0.657137 0.657137 0.695004 0.695004 0.695004 0.730824 0.730824 0.730824 0.764598 0.764598 0.764598 0.796324 0.796324 0.796324 0.826004 0.826004 0.826004 0.853636 0.853636 0.853636 0.879222 0.879222 0.879222 0.902761 0.902761 0.902761 0.924253 0.924253 0.924253 0.943699 0.943699 0.943699 0.961097 0.961097 0.961097 0.976448 0.976448 0.976448 1 1 1 1
  line L65 (-5.5, 66.913) -> (-4.55, 66.913)
  line L66 (-3.8, 69.8) -> (-3.8, 0)
  line L67 (0, 0) -> (-3.8, 0)
  line L68 (0, 69.8) -> (0, 0)
  line L69 (-3.8, 69.8) -> (0, 69.8)
  line L70 (0, 0) -> (-3.8, 0)
  line L71 (-3.8, 0) -> (-4.55, 0)
  line L72 (-4.55, 0) -> (-4.55, 69.8)
  line L73 (-4.55, 69.8) -> (-3.8, 69.8)
  line L74 (-3.8, 69.8) -> (-3.8, 0)
  point P0 (-2.8, 34.8)
  constraints: 8 end point, 2 collinear, 2 parallel, 1 horizontal, 1 perpendicular
extrude "Extrusion5" add sketch "Sketch5" against normal blind 12 contours L2 S1 A0 S0 L1 L0 | L5 S3 A1 S2 L4 L3 | L8 S5 A2 S4 L7 L6 | L63 L65 S43 A21 S42 L64 | L11 S7 A3 S6 L10 L9 | L60 L62 S41 A20 S40 L61 | L14 S9 A4 S8 L13 L12 | L57 L59 S39 A19 S38 L58 | L17 S11 A5 S10 L16 L15 | L54 L56 S37 A18 S36 L55 | L20 S13 A6 S12 L19 L18 | L51 L53 S35 A17 S34 L52 | L23 S15 A7 S14 L22 L21 | L48 L50 S33 A16 S32 L49 | L26 S17 A8 S16 L25 L24 | L45 L47 S31 A15 S30 L46 | L29 S19 A9 S18 L28 L27 | L42 L44 S29 A14 S28 L43 | L32 S21 A10 S20 L31 L30 | L39 L41 S27 A13 S26 L40 | L35 S23 A11 S22 L34 L33 | L36 L38 S25 A12 S24 L37
sketch "Sketch6" plane through (2.8, -21, -34.8) normal (0, -1, 0) x (1, 0, 0)
  line L0 (-3.8, 69.8) -> (-3.8, 0) projected
  line L1 (0, 0) -> (-3.8, 0) projected
  line L2 (0, 69.8) -> (0, 0) projected
  line L3 (-3.8, 69.8) -> (0, 69.8) projected
  line L4 (-4.55, 1.057) -> (-4.55, 2.6868) projected
  line L5 (-4.55, 66.913) -> (-4.55, 68.5428) projected
  line L6 (-3.8, -0.2) -> (0, -0.2) projected
  line L7 (-3.8, 69.8) -> (-3.8, 0) projected
  line L8 (-3.8, 69.8) -> (-4.55, 69.8)
  line L9 (-4.55, 69.8) -> (-4.55, -0.2)
  line L10 (-4.55, -0.2) -> (-3.8, -0.2)
  line L11 (-3.8, -0.2) -> (-3.8, 69.8)
  point P0 (-2.8, 34.8)
  point P1 (-4.55, 2.6868)
  point P2 (-3.8, 0)
  constraints: 8 end point, 2 collinear, 2 parallel, 1 horizontal, 1 perpendicular
extrude "Extrusion6" add sketch "Sketch6" against normal up to surface (14 mm away) contours L0 L11 L10 L9 L4 L5 L8
chamfer "Chamfer5" distance 0.2 angle 45 6 edges at (-1.375, -21, -35) (-1.75, -14, 35) (0.525, -21, 35) (-1.75, -14, -35) (-2.275, -7, -35) (-4.175, -7, 35)
sketch "Sketch7" plane through (0, 0, 35) normal (0, 0, 1) x (1, 0, 0)
  line L0 (-1.55, -6.8) -> (-6.8, -6.8) projected
  line L1 (-1.55, -20.8) -> (-1.55, -6.8) projected
  line L2 (3, -20.8) -> (-1.55, -20.8) projected
  line L3 (3, -20.8) -> (3, -7) projected
  line L4 (3, -7) -> (6.6, -7) projected
  line L5 (6.8, -6.8) -> (6.6, -7) projected
  line L6 (6.8, -6.8) -> (6.8, -0.2) projected
  line L7 (6.6, 0) -> (6.8, -0.2) projected
  line L8 (6.6, 0) -> (3.25, 0) projected
  line L9 (3.25, 0) -> (3.25, 4.6) projected
  line L10 (3.05, 4.8) -> (3.25, 4.6) projected
  line L11 (3.05, 4.8) -> (-3.05, 4.8) projected
  line L12 (-3.25, 4.6) -> (-3.05, 4.8) projected
  line L13 (-3.25, 4.6) -> (-3.25, 0) projected
  line L14 (-3.25, 0) -> (-6.6, 0) projected
  line L15 (-6.8, -0.2) -> (-6.6, 0) projected
  line L16 (-6.8, -0.2) -> (-6.8, -6.8) projected
  line L17 (2.8, -21) -> (-1.75, -21) projected
  line L18 (6.8, -7) -> (1.75, -7)
  line L19 (1.75, -7) -> (1.75, -21)
  line L20 (1.75, -21) -> (6.8, -21)
  line L21 (6.8, -21) -> (6.8, -7)
  point P0 (0, 0)
  point P1 (1.75, -20.8)
  dimension "d47" = 5.05
  constraints: 8 end point, 2 parallel, 2 point on line, 1 collinear, 1 horizontal, 1 perpendicular
  measures "d47" distance of L19.end L20.end
extrude "Extrusion7" cut sketch "Sketch7" against normal through all contours L19 L18 L3 L2 | L2 L3 L4 L18 L21 L20 L17 L19
sketch "Sketch8" plane through (0, 0, 35) normal (0, 0, 1) x (1, 0, 0)
  line L0 (1.75, -20.8) -> (1.75, -7) projected
  line L1 (1.75, -7) -> (6.6, -7) projected
  line L2 (6.8, -6.8) -> (6.6, -7) projected
  line L3 (6.8, -6.8) -> (6.8, -0.2) projected
  line L4 (6.6, 0) -> (6.8, -0.2) projected
  line L5 (6.6, 0) -> (3.25, 0) projected
  line L6 (3.25, 0) -> (3.25, 4.6) projected
  line L7 (3.05, 4.8) -> (3.25, 4.6) projected
  line L8 (3.05, 4.8) -> (-3.05, 4.8) projected
  line L9 (-3.25, 4.6) -> (-3.05, 4.8) projected
  line L10 (-3.25, 4.6) -> (-3.25, 0) projected
  line L11 (-3.25, 0) -> (-6.6, 0) projected
  line L12 (-6.8, -0.2) -> (-6.6, 0) projected
  line L13 (-6.8, -0.2) -> (-6.8, -6.8) projected
  line L14 (-1.55, -6.8) -> (-6.8, -6.8) projected
  line L15 (-1.55, -20.8) -> (-1.55, -6.8) projected
  line L16 (1.75, -20.8) -> (-1.55, -20.8) projected
  line L17 (2.8, -7) -> (1.75, -7) projected
  line L18 (1.75, -7) -> (6.8, -7)
  line L19 (6.8, -7) -> (6.8, 4.8)
  line L20 (6.8, 4.8) -> (1.75, 4.8)
  line L21 (1.75, 4.8) -> (1.75, -7)
  line L22 (6.8, -6.8) -> (6.8, -0.2) projected
  line L23 (3.05, 4.8) -> (-3.05, 4.8) projected
  point P0 (0, 0)
  constraints: 8 end point, 2 collinear, 2 parallel, 1 horizontal, 1 perpendicular
extrude "Extrusion8" cut sketch "Sketch8" against normal through all contours L21 L8 L7 L6 L5 L4 L3 L2 L1
sketch "Sketch9" plane through (0, 0, 35) normal (0, 0, 1) x (1, 0, 0)
  line L0 (1.75, -20.8) -> (1.75, 4.8) projected
  line L1 (1.75, 4.8) -> (-3.05, 4.8) projected
  line L2 (-3.25, 4.6) -> (-3.05, 4.8) projected
  line L3 (-3.25, 4.6) -> (-3.25, 0) projected
  line L4 (-3.25, 0) -> (-6.6, 0) projected
  line L5 (-6.8, -0.2) -> (-6.6, 0) projected
  line L6 (-6.8, -0.2) -> (-6.8, -6.8) projected
  line L7 (-1.55, -6.8) -> (-6.8, -6.8) projected
  line L8 (-1.55, -20.8) -> (-1.55, -6.8) projected
  line L9 (1.75, -20.8) -> (-1.55, -20.8) projected
  line L10 (-6.6, -7) -> (-1.75, -7) projected
  line L11 (1.75, -5.7) -> (1.75, -20.8) projected
  line L12 (1.75, -7) -> (-6.8, -7)
  line L13 (-6.8, -7) -> (-6.8, 4.8)
  line L14 (-6.8, 4.8) -> (1.75, 4.8)
  line L15 (1.75, 4.8) -> (1.75, -7)
  point P0 (0, 0)
  point P1 (-1.55, -7)
  constraints: 8 end point, 3 collinear, 2 parallel, 1 horizontal, 1 perpendicular, 1 point on line
extrude "Extrusion9" cut sketch "Sketch9" against normal through all contours L12 L8 L7 L6 L5 L4 L3 L2 L1 L0 | L12 L10 L13 L7 L8 | L2 L3 L4 L5 L13 L14
equation "\"d15\" = d14"
body "Solid1"
